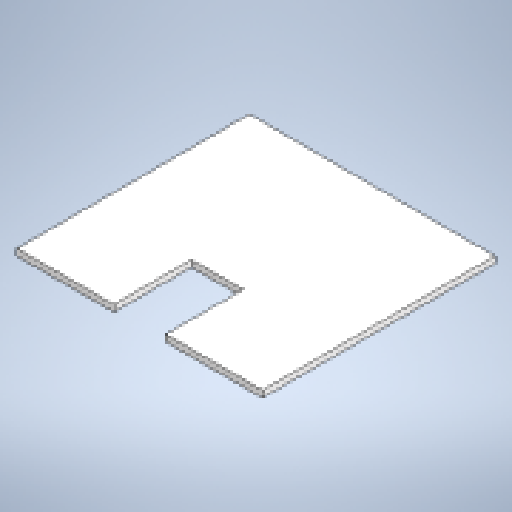
# Autodesk Inventor part: Bottom Plate
Saved by Autodesk Inventor 2023.2 (Build 272271000, 271)
## iProperties
Created: 2023-11-13
Part Number: Bottom Plate
Material: UHMW, White
Document SubType Name: Modeling
Designer: Nathan Cai
Density: 0.94 g/cm^3
Appearance: Smooth - White
Mass: 38.2689 g
Surface Area: 273.79 cm^2
Volume: 40.7116 cm^3
Author: Nathan Cai
Autodesk Inventor part; units mm, degrees
ref_plane "YZ Plane" through (0, 0, 0) normal (1, 0, 0) x (0, 1, 0)
ref_plane "XZ Plane" through (0, 0, 0) normal (0, 1, 0) x (-1, 0, 0)
ref_plane "XY Plane" through (0, 0, 0) normal (0, 0, 1) x (1, 0, 0)
sketch "Sketch1" plane through (0, 0, 0) normal (0, 1, 0) x (-1, 0, 0)
  line L0 (60.325, 57.15) -> (-60.325, 57.15)
  line L1 (-60.325, 57.15) -> (-60.325, -57.15)
  line L2 (-60.325, -57.15) -> (60.325, -57.15)
  line L3 (60.325, -57.15) -> (60.325, 57.15)
  line L4 (60.325, 57.15) -> (-60.325, -57.15) construction
  line L5 (-60.325, 57.15) -> (60.325, -57.15) construction
  line L6 (12.7, 95.25) -> (-12.7, 95.25)
  line L7 (-12.7, 95.25) -> (-12.7, 19.05)
  line L8 (-12.7, 19.05) -> (12.7, 19.05)
  line L9 (12.7, 19.05) -> (12.7, 95.25)
  line L10 (12.7, 95.25) -> (-12.7, 19.05) construction
  line L11 (-12.7, 95.25) -> (12.7, 19.05) construction
  point P0 (0, 0)
  point P1 (0, 57.15)
  point P2 (12.7, 57.15)
  point P3 (-12.7, 57.15)
  dimension "d0" = 120.65
  dimension "d1" = 114.3
  dimension "d2" = 25.4
  dimension "d3" = 76.2
  constraints: 24 end point, 5 midpoint, 4 parallel, 2 horizontal, 2 perpendicular
  measures "d0" distance of L2.end L1.end
  measures "d1" distance of L1.end L0.end
  measures "d2" distance of L8.end L7.end
  measures "d3" distance of L7.end L6.end
extrude "Extrusion1" add sketch "Sketch1" along normal blind 3.175 contours L3 L2 L1 L0 L7 L8 L9
body "Solid1"
